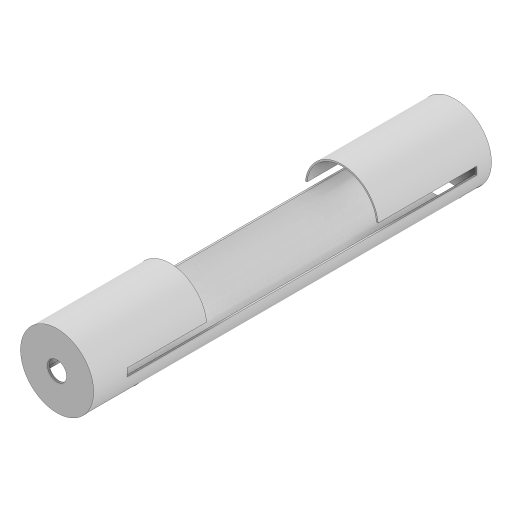
# Autodesk Inventor part: GUIA_DE_OBJETO
Saved by Autodesk Inventor 2024 (Build 280153000, 153)
## iProperties
Created: 2024-05-26
Part Number: GUIA_DE_OBJETO
Material: Generic
Document SubType Name: Modeling
Designer: Jhuliams
Density: 1 g/cm^3
Appearance: Default
Author: Jhuliams
Autodesk Inventor part; units mm, degrees
ref_plane "YZ Plane" through (0, 0, 0) normal (1, 0, 0) x (0, 1, 0)
ref_plane "XZ Plane" through (0, 0, 0) normal (0, 1, 0) x (-1, 0, 0)
ref_plane "XY Plane" through (0, 0, 0) normal (0, 0, 1) x (1, 0, 0)
sketch "Sketch1" plane through (0, 0, 0) normal (0, 0, 1) x (1, 0, 0)
  circle A0 centre (0, 0) radius 57.5
  line L0 (-57.5, 0) -> (57.5, 0)
  circle A1 centre (0, 0) radius 55
  point P0 (55, 0)
  point P1 (-55, 0)
  dimension "d0" = 115
  dimension "d2" = 110
  constraints: 2 centre point, 2 coincident, 2 end point, 2 point on circle, 1 horizontal
  measures "d0" diameter of A0
  measures "d2" diameter of A1
extrude "Extrusion1" add sketch "Sketch1" along normal mid plane 620 contours L0 A1 A0 | A0 L0 A1
sketch "Sketch3" plane through (0, 0, 310) normal (0, 0, 1) x (1, 0, 0)
  circle A0 centre (0, 0) radius 57.5
  dimension "d5" = 115
  constraints: 1 centre point, 1 coincident
  measures "d5" diameter of A0
extrude "Extrusion2" add sketch "Sketch3" along normal blind 3
sketch "Sketch4" plane through (0, 0, -310) normal (0, 0, -1) x (-1, 0, 0)
  circle A0 centre (0, 0) radius 57.5
  dimension "d8" = 115
  constraints: 1 centre point, 1 coincident
  measures "d8" diameter of A0
extrude "Extrusion3" add sketch "Sketch4" along normal blind 3
sketch "Sketch5" plane through (0, 0, 0) normal (0, 1, 0) x (-1, 0, 0)
  line L0 (0, 0) -> (0, 270) construction
  line L1 (45, 310) -> (-45, 310)
  line L2 (-45, 310) -> (-45, 230)
  line L3 (-45, 230) -> (45, 230)
  line L4 (45, 230) -> (45, 310)
  line L5 (45, 310) -> (-45, 230) construction
  line L6 (-45, 310) -> (45, 230) construction
  line L7 (0, 0) -> (20, 0) construction
  line L8 (0, 0) -> (0, -295)
  line L9 (-45, -280) -> (45, -280)
  line L10 (45, -280) -> (45, -310)
  line L11 (45, -310) -> (-45, -310)
  line L12 (-45, -310) -> (-45, -280)
  line L13 (-45, -280) -> (45, -310) construction
  line L14 (45, -280) -> (-45, -310) construction
  dimension "d11" = 270
  dimension "d12" = 90
  dimension "d13" = 80
  dimension "d14" = 20
  dimension "d37" = 295
  dimension "d38" = 90
  dimension "d39" = 30
  constraints: 30 end point, 4 midpoint, 4 parallel, 3 horizontal, 2 perpendicular, 2 vertical
  measures "d11" distance of L0.start L0.end
  measures "d12" distance of L3.end L2.end
  measures "d13" distance of L2.end L1.end
  measures "d14" distance of L0.start L7.end
  measures "d37" distance of L0.start L8.end
  measures "d38" distance of L10.end L11.end
  measures "d39" distance of L9.end L10.end
extrude "Extrusion4" cut sketch "Sketch5" against normal blind 80
sketch "Sketch6" plane through (0, 0, 0) normal (0, 1, 0) x (-1, 0, 0)
  line L0 (60, 135) -> (-60, 135)
  line L1 (-60, 135) -> (-60, -135)
  line L2 (-60, -135) -> (60, -135)
  line L3 (60, -135) -> (60, 135)
  line L4 (60, 135) -> (-60, -135) construction
  line L5 (-60, 135) -> (60, -135) construction
  point P0 (0, 0)
  dimension "d17" = 120
  dimension "d18" = 270
  constraints: 12 end point, 2 midpoint, 2 parallel, 1 horizontal, 1 perpendicular
  measures "d17" distance of L2.end L1.end
  measures "d18" distance of L1.end L0.end
extrude "Extrusion5" cut sketch "Sketch6" along normal blind 100
sketch "Sketch7" plane through (0, 0, 0) normal (1, 0, 0) x (0, 1, 0)
  line L0 (6, 280) -> (-6, 280)
  line L1 (-6, 280) -> (-6, -280)
  line L2 (-6, -280) -> (6, -280)
  line L3 (6, -280) -> (6, 280)
  line L4 (6, 280) -> (-6, -280) construction
  line L5 (-6, 280) -> (6, -280) construction
  line L6 (-6, 0) -> (6, 0)
  line L7 (6, 0) -> (-6, 0)
  line L8 (-6, 0) -> (-6, -290)
  line L9 (-6, -290) -> (6, -290)
  line L10 (6, -290) -> (6, 0)
  line L11 (6, 0) -> (-6, 0)
  line L12 (-6, 0) -> (-6, 260)
  line L13 (-6, 260) -> (6, 260)
  line L14 (6, 260) -> (6, 0)
  point P0 (0, 0)
  point P1 (6, 260)
  point P2 (-6, 260)
  dimension "d21" = 12
  dimension "d22" = 560
  dimension "d34" = 290
  dimension "d35" = 12
  dimension "d36" = 260
  constraints: 30 end point, 6 parallel, 4 midpoint, 3 horizontal, 3 perpendicular
  measures "d21" distance of L2.end L1.end
  measures "d22" distance of L1.end L0.end
  measures "d34" distance of L8.end L7.end
  measures "d35" distance of L12.end L13.end
  measures "d36" distance of L11.end L12.end
extrude "Extrusion6" cut sketch "Sketch7" along normal mid plane 200 contours L3 L6 L1 L13 | L3 L2 L1 L6 | L10 L9 L8 L2
sketch "Sketch8" plane through (0, 0, 313) normal (0, 0, 1) x (1, 0, 0)
  circle A0 centre (0, 0) radius 15
  dimension "d25" = 30
  constraints: 1 centre point, 1 coincident
  measures "d25" diameter of A0
extrude "Extrusion7" cut sketch "Sketch8" against normal blind 1000
body "Solid1"
